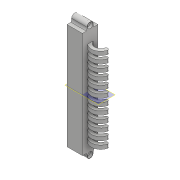
# Autodesk Inventor part: Part1
Saved by Autodesk Inventor 2017 (Build 210142000, 142)
## iProperties
Created: 2019-09-23
Part Number: Part1
Material: Generic
Document SubType Name: Modeling
Designer: Admin
Density: 1 g/cm^3
Appearance: Default
Author: Admin
Autodesk Inventor part; units mm, degrees
ref_plane "YZ Plane" through (0, 0, 0) normal (1, 0, 0) x (0, 1, 0)
ref_plane "XZ Plane" through (0, 0, 0) normal (0, 1, 0) x (-1, 0, 0)
sketch "Sketch1" plane through (0, 0, 0) normal (0, 0, 1) x (1, 0, 0)
  line L0 (0, 0) -> (-250, 0)
  line L1 (-250, 0) -> (-250, 250)
  line L2 (-250, 250) -> (0, 250)
  line L3 (0, 250) -> (0, 0)
  line L4 (-63.1596, 186.8404) -> (-186.8404, 186.8404)
  line L5 (-186.8404, 186.8404) -> (-186.8404, 63.1596)
  line L6 (-186.8404, 63.1596) -> (-63.1596, 63.1596)
  line L7 (-63.1596, 63.1596) -> (-63.1596, 186.8404)
  dimension "d0" = 250
  dimension "d1" = 250
  constraints: 16 end point, 4 parallel, 2 perpendicular, 1 horizontal, 3 other
  measures "d0" distance of L1.end L2.end
  measures "d1" distance of L0.end L1.end
extrude "Extrusion1" add sketch "Sketch1" along normal blind 1720
ref_plane "Work Plane1" through (0, 0, 1645) normal (0, 0, 1) x (1, 0, 0)
sketch "Sketch2" plane through (0, 0, 1645) normal (0, 0, 1) x (1, 0, 0)
  line L0 (0, 0) -> (0, 250) projected
  arc A0 (0, 176.8241) -> (194.6786, 176.8241) centre (97.3393, 201.2611) ccw
  arc A1 (-52.0326, 163.7613) -> (246.7111, 163.7613) centre (97.3393, 201.2611) ccw
  arc A2 (246.7111, 163.7613) -> (194.6786, 176.8241) centre (219.3741, 165.032) ccw
  line L1 (0, 176.8241) -> (0, 81.916)
  constraints: 7 point on circle, 3 centre point, 2 end point, 2 point on line
extrude "Extrusion2" add sketch "Sketch2" against normal blind 60.5 separate body
pattern_linear "Rectangular Pattern1" count 14 spacing 120 along (0, 0, -1) of "Extrusion2" bodies 2
sketch "Sketch3" plane through (-250, 0, 0) normal (-1, 0, 0) x (0, 0, 1)
  line L0 (1720, 63.1596) -> (1720, 186.8404) projected
  line L1 (1720, 125) -> (1820, 125)
  circle A0 centre (1770, 125) radius 50
  circle A1 centre (1770, 125) radius 45.2836
  arc A2 (1720, 186.8404) -> (1769.4702, 174.9972) centre (1768.3617, 279.6092) ccw
  line L2 (0, 63.1596) -> (1720, 63.1596) projected
  arc A3 (1769.4702, 75.0028) -> (1720, 63.1596) centre (1760.5864, 2.8687) ccw
  line L3 (1720, 186.8404) -> (1720, 63.1596)
  point P0 (0, 0)
  dimension "d10" = 100
  constraints: 7 point on circle, 4 centre point, 4 end point, 2 midpoint, 1 coincident, 1 horizontal, 1 tangent, 1 vertical
  measures "d10" distance of L1.start L1.end
extrude "Extrusion3" add sketch "Sketch3" against normal blind 250 separate body contours L0 A0 A3 | A0 L1 A1 | L0 A2 A0 | L1 A1 A0 A3
ref_plane "Work Plane2" through (0, 0, 860) normal (0, 0, -1) x (-1, 0, 0)
mirror "Mirror1" about plane through (0, 0, 860) normal (0, 0, -1) of "Extrusion3" bodies 3
sketch "Sketch4" plane through (-250, 0, 0) normal (-1, 0, 0) x (0, 0, 1)
  line L0 (553.261, 250) -> (553.261, 386.8741)
  line L1 (553.261, 386.8741) -> (1166.739, 386.8741)
  line L2 (1166.739, 386.8741) -> (1166.739, 250)
  line L3 (0, 250) -> (1720, 250) projected
  line L4 (1166.739, 113.1259) -> (553.261, 386.8741) construction
  line L5 (553.261, 113.1259) -> (1166.739, 386.8741) construction
  line L6 (553.261, 250) -> (1166.739, 250)
  line L7 (1720, 63.1596) -> (1720, 186.8404) projected
  line L8 (1720, 125) -> (1656.5062, 125)
  line L9 (553.261, 0) -> (553.261, -136.8741)
  line L10 (553.261, -136.8741) -> (1166.739, -136.8741)
  line L11 (1166.739, -136.8741) -> (1166.739, 0)
  line L12 (0, 0) -> (1720, 0)
  point P0 (860, 250)
  constraints: 22 end point, 6 symmetric about line, 4 midpoint, 4 point on line, 1 horizontal, 1 parallel
extrude "Extrusion4" add sketch "Sketch4" along normal blind 4000 and the other way blind 112.625 bodies 1
sketch "Sketch5" plane through (-4250, 0, 0) normal (-1, 0, 0) x (0, 0, 1)
  line L0 (553.261, 250) -> (553.261, 386.8741) projected
  line L1 (1166.739, -136.8741) -> (553.261, -136.8741) projected
  line L2 (553.261, 386.8741) -> (1166.739, 386.8741)
  line L3 (1166.739, 386.8741) -> (1166.739, -136.8741)
  line L4 (1166.739, -136.8741) -> (553.261, -136.8741)
  line L5 (553.261, -136.8741) -> (553.261, 386.8741)
  point P0 (0, 0)
  constraints: 8 end point, 2 parallel, 1 horizontal, 1 perpendicular
extrude "Extrusion5" add sketch "Sketch5" along normal blind 313.75 bodies 1
sketch "Sketch6" plane through (-4250, 0, 1166.739) normal (0, 0, 1) x (1, 0, 0)
  line L0 (0, 0) -> (4000, 0) projected
  line L1 (4000, 0) -> (2000, 0)
  line L2 (4000, 250) -> (0, 250) projected
  line L3 (1981.6419, 0) -> (1582.3554, 0)
  line L4 (1582.3554, 0) -> (1582.3554, 250)
  line L5 (1582.3554, 250) -> (1981.6419, 250)
  line L6 (1981.6419, 250) -> (1981.6419, 0)
  point P0 (4250, 0)
  dimension "d19" = 2000
  constraints: 10 end point, 2 parallel, 2 point on line, 1 horizontal, 1 midpoint, 1 perpendicular
  measures "d19" distance of L0.end L1.end
extrude "Extrusion6" add sketch "Sketch6" along normal blind 443.75 and the other way blind 968.125 separate body
move faces "Move1" translate (-4000, 0, 0) faces at (-137.375, 341.2494, 757.7537)
move faces "Move2" translate (-4000, 0, 0) faces at (-137.375, -45.6247, 757.7537)
sketch "Sketch7" plane through (-4563.75, 386.8741, 1166.739) normal (0, 1, 0) x (1, 0, 0)
  line L0 (-160.429, 1507.8096) -> (2898.7777, 1507.8096)
  line L1 (2898.7777, 1507.8096) -> (2898.7777, -823.903)
  line L2 (2898.7777, -823.903) -> (-160.429, -823.903)
  line L3 (-160.429, -823.903) -> (-160.429, 1507.8096)
  point P0 (4563.75, 1166.739)
  constraints: 8 end point, 2 parallel, 1 horizontal, 1 perpendicular
extrude "Extrusion7" cut sketch "Sketch7" against normal blind 1321 bodies 1
sketch "Sketch8" plane through (-2667.6446, 250, 1610.489) normal (0, 1, 0) x (1, 0, 0)
  line L0 (-207.7162, 1776.1272) -> (939.481, 1776.1272)
  line L1 (939.481, 1776.1272) -> (939.481, -698.7251)
  line L2 (939.481, -698.7251) -> (-207.7162, -698.7251)
  line L3 (-207.7162, -698.7251) -> (-207.7162, 1776.1272)
  point P0 (2667.6446, 1610.489)
  constraints: 8 end point, 2 parallel, 1 horizontal, 1 perpendicular
extrude "Extrusion8" cut sketch "Sketch8" against normal blind 1280.5 bodies 4
sketch "Sketch9" plane through (-250, 125, -50) normal (-1, 0, 0) x (0, 0, 1)
  circle A0 centre (0, 0) radius 45.2836 projected
  circle A1 centre (0, 0) radius 45.2836
  point P0 (50, -125)
  constraints: 1 centre point, 1 coincident, 1 concentric
extrude "Extrusion9" add sketch "Sketch9" against normal blind 210 bodies 3
sketch "Sketch10" plane through (-250, 0, 0) normal (-1, 0, 0) x (0, 0, 1)
  circle A0 centre (1770, 125) radius 45.2836 projected
  circle A1 centre (1770, 125) radius 45.2836
  point P0 (0, 0)
  constraints: 1 centre point, 1 coincident, 1 concentric
extrude "Extrusion10" add sketch "Sketch10" against normal blind 210 bodies 3
move faces "Move3" translate (0, 0, 62.25) faces at (45.5046, 75.6082, 24.5) (15.5333, 143.1244, 64.8333)
move faces "Move4" translate (0, 0, -75) faces at (45.5046, 75.6082, 1645)
combine bodies "Combine1" operation type add bodies to combine 1 2 3 4
body "Solid4"
